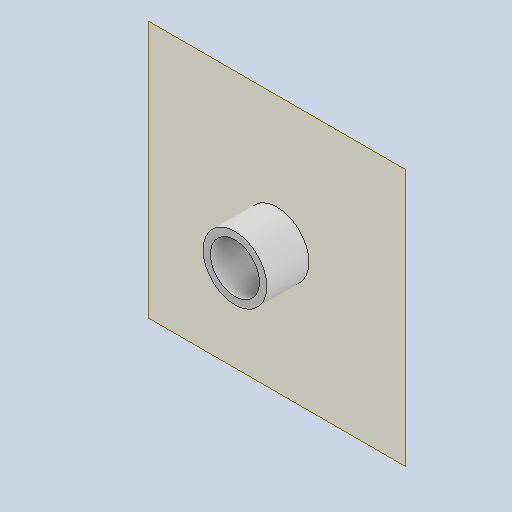
# Autodesk Inventor part: стакан
Saved by Autodesk Inventor 2023 (Build 270158000, 158)
## iProperties
Created: 2025-02-03
Part Number: стакан
Material: Типовые
Document SubType Name: Modeling
Designer: baranovaem
Density: 1 g/cm^3
Appearance: По умолчанию
Author: baranovaem
Autodesk Inventor part; units mm, degrees
ref_plane "YZ Plane" through (0, 0, 0) normal (1, 0, 0) x (0, 1, 0)
ref_plane "XZ Plane" through (0, 0, 0) normal (0, 1, 0) x (-1, 0, 0)
ref_plane "РабПлоскость1" through (0, 0, 0) normal (0, 0, 1) x (1, 0, 0)
sketch "Эскиз1" plane through (0, 0, 0) normal (0, 0, 1) x (1, 0, 0)
  circle A0 centre (0, 0) radius 10
  circle A1 centre (0, 0) radius 13
  dimension "d0" = 20
  dimension "d1" = 26
  constraints: 2 centre point, 2 coincident
  measures "d0" diameter of A0
  measures "d1" diameter of A1
ref_plane "РабПлоскость2" through (-114.5188, -114.5187, 17.2192) normal (0, 0, -1) x (0.437, 0.8995, 0)
extrude "Выдавливание1" add sketch "Эскиз1" along normal up to surface (17.2192 mm away)
